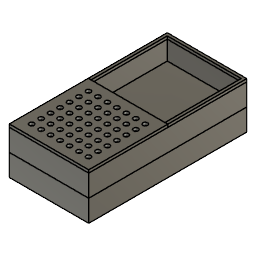
car-chassis-v1 (Autodesk Fusion 360 design; units mm, degrees)
part number: 2026-07-21-18-30-28-166
Autodesk Fusion 360 part; units mm, degrees
sketch "Sketch1" plane through (0, 0, 0) normal (0, 0, 1) x (1, 0, 0)
  line L0 (42, -83.5) -> (-42, -83.5)
  line L1 (-42, -83.5) -> (-42, 83.5)
  line L2 (-42, 83.5) -> (42, 83.5)
  line L3 (42, 83.5) -> (42, -83.5)
  line L4 (42, -83.5) -> (-42, 83.5) construction
  line L5 (-42, -83.5) -> (42, 83.5) construction
  dimension "d7" = 84
  dimension "d8" = 167
  constraint horizontal L0
  constraint perpendicular L0 L1
  constraint parallel L0 L2
  constraint parallel L1 L3
  constraint coincident L4 origin
  constraint coincident L5 origin
  measures "d7" distance of L1.end L2.end
  measures "d8" distance of L0.start L2.end
extrude "Extrude1" add sketch "Sketch1" along normal blind 3 makes body 1
ref_plane "WorkPlane1" through (0, 0, 1.5) normal (0, 1, 0) x (-1, 0, 0)
ref_plane "WorkPlane2" through (0, 0, 1.5) normal (1, 0, 0) x (0, 1, 0)
sketch "Sketch2" plane through (42, 0, 0) normal (1, 0, 0) x (0, 1, 0)
  line L0 (-83.5, 0) -> (83.5, 0)
  line L1 (83.5, 0) -> (83.5, 3)
  line L2 (83.5, 3) -> (-83.5, 3)
  line L3 (-83.5, 3) -> (-83.5, 0)
  line L4 (-83.5, 3) -> (83.5, 3)
  line L5 (83.5, 3) -> (83.5, 23)
  line L6 (83.5, 23) -> (-83.5, 23)
  line L7 (-83.5, 23) -> (-83.5, 3)
  dimension "d12" = 167
  dimension "d13" = 20
  constraint horizontal L4
  constraint vertical L5
  constraint horizontal L6
  constraint vertical L7
  constraint coincident L2.end L3.start
  measures "d12" distance of L5.end L6.end
  measures "d13" distance of L1.end L5.end
extrude "Extrude2" add sketch "Sketch2" against normal blind 3 separate body contours L2 L4 L5 L6 L7 makes body 2
mirror "Mirror1" about plane through (0, 0, 1.5) normal (1, 0, 0) of bodies 2 makes body 3
sketch "Sketch3" plane through (0, -83.5, 0) normal (0, -1, 0) x (1, 0, 0)
  line L0 (-42, 0) -> (42, 0)
  line L1 (42, 0) -> (42, 3)
  line L2 (42, 3) -> (-42, 3)
  line L3 (-42, 3) -> (-42, 0)
  line L4 (-42, 3) -> (42, 3)
  line L5 (42, 3) -> (42, 23)
  line L6 (42, 23) -> (-42, 23)
  line L7 (-42, 23) -> (-42, 3)
  dimension "d18" = 84
  dimension "d19" = 20
  constraint horizontal L4
  constraint vertical L5
  constraint horizontal L6
  constraint vertical L7
  constraint coincident L2.end L3.start
  measures "d18" distance of L5.end L6.end
  measures "d19" distance of L1.end L5.end
extrude "Extrude3" cut sketch "Sketch3" against normal blind 3 contours L2 L4 L5 L6 L7 bodies 2 3
sketch "Sketch4" plane through (0, -83.5, 0) normal (0, -1, 0) x (1, 0, 0)
  line L0 (-42, 0) -> (42, 0)
  line L1 (42, 0) -> (42, 3)
  line L2 (42, 3) -> (-42, 3)
  line L3 (-42, 3) -> (-42, 0)
  line L4 (-42, 3) -> (42, 3)
  line L5 (42, 3) -> (42, 23)
  line L6 (42, 23) -> (-42, 23)
  line L7 (-42, 23) -> (-42, 3)
  dimension "d22" = 20
  dimension "d23" = 84
  constraint horizontal L4
  constraint vertical L5
  constraint horizontal L6
  constraint vertical L7
  constraint coincident L2.end L3.start
  measures "d22" distance of L1.end L5.end
  measures "d23" distance of L5.end L6.end
extrude "Extrude4" add sketch "Sketch4" against normal blind 3 separate body contours L2 L4 L5 L6 L7 makes body 4
sketch "Sketch5" plane through (0, 83.5, 0) normal (0, 1, 0) x (-1, 0, 0)
  line L0 (-42, 0) -> (42, 0)
  line L1 (42, 0) -> (42, 3)
  line L2 (42, 3) -> (-42, 3)
  line L3 (-42, 3) -> (-42, 0)
  line L4 (-42, 3) -> (42, 3)
  line L5 (42, 3) -> (42, 23)
  line L6 (42, 23) -> (-42, 23)
  line L7 (-42, 23) -> (-42, 3)
  dimension "d26" = 84
  dimension "d27" = 20
  constraint horizontal L4
  constraint vertical L5
  constraint horizontal L6
  constraint vertical L7
  constraint coincident L2.end L3.start
  measures "d26" distance of L5.end L6.end
  measures "d27" distance of L1.end L5.end
extrude "Extrude5" cut sketch "Sketch5" against normal blind 3 contours L2 L4 L5 L6 L7 bodies 2 3
mirror "Mirror2" about plane through (0, 0, 1.5) normal (0, 1, 0) of bodies 4 makes body 5
combine "Combine1" operation add target body 2 tool bodies 5
combine "Combine2" operation add target body 3 tool bodies 2
combine "Combine3" operation add target body 3 tool bodies 4
combine "Combine4" operation add target body 1 tool bodies 3
copy_body "CopyPasteBodies1" bodies 1 makes body 6
move_body "Move1" bodies 6 to x (1, 0, 0) y (0, 1, 0) z (0, 0, 1) at (0, 0, 23)
sketch "Sketch6" plane through (0, 0, 46) normal (0, 0, 1) x (-1, 0, 0)
  line L0 (-42, 83.5) -> (-42, -83.5)
  line L1 (-42, -83.5) -> (42, -83.5)
  line L2 (42, -83.5) -> (42, 83.5)
  line L3 (42, 83.5) -> (-42, 83.5)
  line L4 (-39, 80.5) -> (39, 80.5)
  line L5 (39, 80.5) -> (39, -80.5)
  line L6 (39, -80.5) -> (-39, -80.5)
  line L7 (-39, -80.5) -> (-39, 80.5)
  line L8 (42, 83.5) -> (-42, 83.5)
  line L9 (-42, 83.5) -> (-42, 0)
  line L10 (-42, 0) -> (42, 0)
  line L11 (42, 0) -> (42, 83.5)
  dimension "d32" = 84
  dimension "d33" = 83.5
  constraint horizontal L8
  constraint vertical L9
  constraint horizontal L10
  constraint vertical L11
  constraint coincident L2.end L3.start
  measures "d32" distance of L9.end L10.end
  measures "d33" distance of L0.start L9.end
extrude "Extrude6" add sketch "Sketch6" along normal blind 3 separate body contours L0 L2 L3 L4 L5 L7 L8 L9 L10 L11 | L4 L5 L7 L10 makes body 7
ref_plane "WorkPlane3" through (0, -41.75, 47.5) normal (0, 1, 0) x (-1, 0, 0)
sketch "Sketch7" plane through (0, 0, 49) normal (0, 0, 1) x (-1, 0, 0)
  line L0 (42, 0) -> (42, 83.5)
  line L1 (42, 83.5) -> (-42, 83.5)
  line L2 (-42, 83.5) -> (-42, 0)
  line L3 (-42, 0) -> (42, 0)
  circle A0 centre (0, 41.75) radius 2.5
  dimension "d37" = 5
  measures "d37" diameter of A0
extrude "Extrude7" cut sketch "Sketch7" against normal blind 3 contours A0 bodies 7
pattern_linear "R-Pattern1" count 7 spacing 10 along (0, 1, 0) both ways count 7 spacing 10 along (1, 0, 0) both ways of "Extrude7"
ref_plane "WorkPlane4" through (0, 0, 34.5) normal (0, -1, 0) x (1, 0, 0)
split_face "SplitFace1" 1 faces at (41, -26.8333, 46) by plane through (0, 0, 34.5) normal (0, -1, 0) on bodies 6
extrude "Extrude8" add 1 faces at (13, 82.5, 46) along direction (0, 0, 1) blind 3 separate body on bodies 6 makes body 8
equation "wall = 3 mm" comment "Wall thickness"
equation "clearance = 2 mm" comment "Component to wall gap"
equation "chassis_width = 84 mm" comment "External width"
equation "chassis_length = 167 mm" comment "External length"
equation "d7 = chassis_width"
equation "d8 = chassis_length"
equation "d9 = wall"
equation "tier_height = 20 mm" comment "The height of each tier/wall without including the base"
equation "d12 = chassis_length"
equation "d13 = tier_height"
equation "d14 = -wall"
equation "d18 = chassis_width"
equation "d19 = tier_height"
equation "d20 = -wall"
equation "d22 = tier_height"
equation "d23 = chassis_width"
equation "d24 = -wall"
equation "d26 = chassis_width"
equation "d27 = tier_height"
equation "d28 = -wall"
equation "d32 = chassis_width"
equation "d33 = chassis_length / 2"
equation "d34 = wall"
equation "hole = 5 mm" comment "hole size"
equation "d37 = hole"
equation "d38 = -wall"
equation "d42 = hole * 2"
equation "d43 = hole * 2"
equation "d44 = wall"
